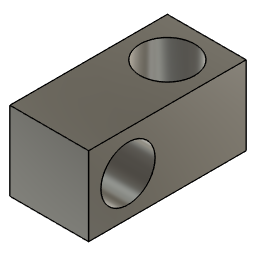
joint_revised (Autodesk Fusion 360 design; units mm, degrees)
Autodesk Fusion 360 part; units mm, degrees
sketch "スケッチ1" plane through (0, 0, 0) normal (0, 0, 1) x (1, 0, 0)
  line L0 (0, 0) -> (-8, 0)
  line L1 (-8, 0) -> (-8, 16)
  line L2 (-8, 16) -> (0, 16)
  line L3 (0, 16) -> (0, 0)
  dimension "d1" = 8
  dimension "d2" = 16
  constraint horizontal L0
  constraint vertical L1
  constraint horizontal L2
  constraint vertical L3
  constraint coincident L0.start L3.end
  measures "d1" distance of L0.start L0.end
  measures "d2" distance of L0.start L2.end
extrude "押し出し1" add sketch "スケッチ1" along normal blind 8
sketch "スケッチ2" plane through (0, 0, 0) normal (1, 0, 0) x (0, 1, 0)
  line L0 (0, 0) -> (16, 0)
  line L1 (16, 0) -> (16, 8)
  line L2 (16, 8) -> (0, 8)
  line L3 (0, 8) -> (0, 0)
  point P0 (4, 4)
  dimension "d5" = 4
  dimension "d6" = 4
  measures "d5" distance of L3 P0
  measures "d6" distance of L0 P0
hole "穴1" at (0, 4, 4) direction (-1, 0, 0) diameter 5.5 depth 10 tip angle 118
sketch "スケッチ3" plane through (0, 0, 8) normal (0, 0, 1) x (-1, 0, 0)
  line L0 (0, -16) -> (8, -16)
  line L1 (8, -16) -> (8, 0)
  line L2 (8, 0) -> (0, 0)
  line L3 (0, 0) -> (0, -16)
  point P0 (4, -12)
  dimension "d10" = 4
  dimension "d11" = 4
  measures "d10" distance of L0 P0
  measures "d11" distance of L1 P0
hole "穴2" at (-4, 12, 8) direction (0, 0, -1) diameter 5.55 depth 10 tip angle 118
